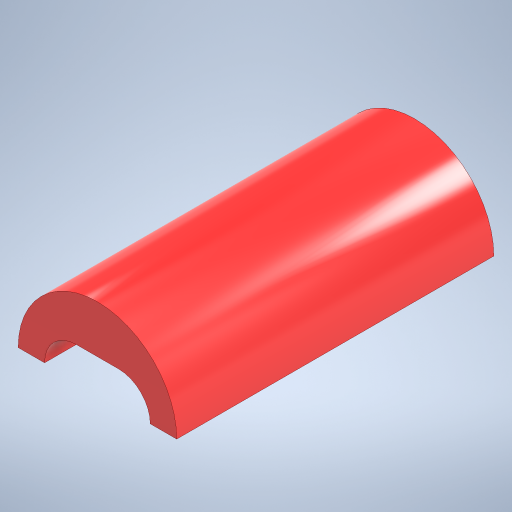
# Autodesk Inventor part: TPU_FootGrip
Saved by Autodesk Inventor 2024 (Build 280153000, 153)
## iProperties
Created: 2024-06-05
Part Number: TPU_FootGrip
Material: Generic
Document SubType Name: Modeling
Designer: Hemant
Density: 1 g/cm^3
Appearance: Light Red
Author: Hemant
Autodesk Inventor part; units mm, degrees
ref_plane "YZ Plane" through (0, 0, 0) normal (1, 0, 0) x (0, 1, 0)
ref_plane "XZ Plane" through (0, 0, 0) normal (0, 1, 0) x (-1, 0, 0)
ref_plane "XY Plane" through (0, 0, 0) normal (0, 0, 1) x (1, 0, 0)
sketch "Sketch1" plane through (0, 0, 0) normal (0, 0, 1) x (1, 0, 0)
  circle A0 centre (0, 4.5) radius 5 construction
  arc A1 (5, 4.5) -> (2, 7.5) centre (2, 4.5) ccw
  line L0 (-2, 7.5) -> (2, 7.5)
  line L1 (-5, 4.5) -> (5, 4.5) construction
  arc A2 (7.5, 4.5) -> (-7.5, 4.5) centre (0, 4.5) ccw
  line L2 (-5, 4.5) -> (-7.5, 4.5)
  line L3 (5, 4.5) -> (7.5, 4.5)
  arc A3 (-2, 7.5) -> (-5, 4.5) centre (-2, 4.5) ccw
  line L4 (0, 0) -> (11.6743, 0) construction
  dimension "d0" = 10
  dimension "d2" = 6
  dimension "d3" = 4
  dimension "d4" = 10
  dimension "d5" = 15
  dimension "d14" = 3
  dimension "d15" = 4.5
  constraints: 10 end point, 6 point on circle, 5 horizontal, 4 centre point, 3 coincident, 1 horizontal alignment, 1 midpoint, 1 point on line, 1 tangent
  measures "d0" diameter of A0
  measures "d2" diameter of A1
  measures "d3" distance of L0.end L0.start
  measures "d4" distance of L1.start L1.end
  measures "d5" diameter of A2
  measures "d14" distance from line of point (0, 4.5) L0
  measures "d15" distance between parallel lines of L4 L1
extrude "Extrusion1" add sketch "Sketch1" along normal blind 30
sketch "Sketch2" plane through (-2, 7.5, 0) normal (0, -1, 0) x (1, 0, 0)
  circle A0 centre (2, 25) radius 1
  circle A1 centre (2, 5) radius 1
  line L0 (0, 30) -> (4, 30) projected
  line L1 (0, 0) -> (4, 0) projected
  point P0 (2, 0)
  point P1 (2, 0)
  point P2 (2, 0)
  dimension "d8" = 2
  dimension "d9" = 2
  dimension "d10" = 5
  dimension "d11" = 5
  constraints: 2 centre point, 2 midpoint, 2 vertical alignment
  measures "d8" diameter of A0
  measures "d9" diameter of A1
  measures "d10" distance from line of L0 A0.centre
  measures "d11" distance of point (2, 0) A1.centre
extrude "Extrusion2" add sketch "Sketch2" along normal blind 3
body "Solid1"
